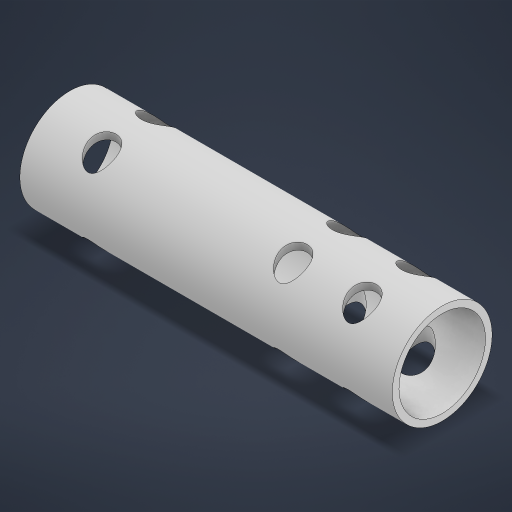
# Autodesk Inventor part: ArmSupportSteelTubing
Saved by Autodesk Inventor 2024 (Build 280153000, 153)
## iProperties
Created: 2024-02-23
Part Number: ArmSupportSteelTubing
Material: Generic
Document SubType Name: Modeling
Designer: avsar
Density: 1 g/cm^3
Appearance: Default
Author: avsar
Autodesk Inventor part; units mm, degrees
ref_plane "YZ Plane" through (0, 0, 0) normal (1, 0, 0) x (0, 1, 0)
ref_plane "XZ Plane" through (0, 0, 0) normal (0, 1, 0) x (-1, 0, 0)
sketch "Sketch1" plane through (0, 0, 0) normal (1, 0, 0) x (0, 1, 0)
  circle A0 centre (0, 0) radius 6.5
  circle A1 centre (0, 0) radius 7.5
  dimension "d0" = 13
  dimension "d1" = 15
  constraints: 2 centre point, 2 coincident
  measures "d0" diameter of A0
  measures "d1" diameter of A1
extrude "Extrusion1" add sketch "Sketch1" along normal blind 56
sketch "Sketch2" plane through (56, 0, 0) normal (1, 0, 0) x (0, 0, -1)
  circle A0 centre (0, 0) radius 7.5 construction
  line L0 (0, 7.5) -> (0, -7.5)
  constraints: 2 end point, 2 point on circle, 1 midpoint, 1 vertical
ref_plane "Work Plane1" through (56, 7.5, 0) normal (0, 1, 0) x (-1, 0, 0)
sketch "Sketch3" plane through (56, 7.5, 0) normal (0, 1, 0) x (-1, 0, 0)
  circle A0 centre (8, -4) radius 2.1
  circle A1 centre (8, 4) radius 2.1
  line L0 (8, 4) -> (8, -4) construction
  line L1 (56, -7.5) -> (0, -7.5) construction
  line L2 (28, -7.5) -> (28, 7.5) construction
  line L3 (56, 7.5) -> (0, 7.5) construction
  line L4 (12.75, 7.5) -> (3.25, 7.5) construction
  line L5 (3.25, 7.5) -> (3.25, -7.5) construction
  line L6 (3.25, -7.5) -> (12.75, -7.5) construction
  line L7 (12.75, -7.5) -> (12.75, 7.5) construction
  line L8 (12.75, 7.5) -> (3.25, -7.5) construction
  line L9 (3.25, 7.5) -> (12.75, -7.5) construction
  line L10 (13.2, -7.5) -> (13.2, 7.5) construction
  circle A2 centre (18.4, -4) radius 2.1
  circle A3 centre (18.4, 4) radius 2.1
  circle A4 centre (47.15, -4) radius 2.1
  circle A5 centre (47.15, 4) radius 2.1
  line L11 (47.15, -4) -> (47.15, 4)
  point P0 (56, 0)
  point P1 (28, 0)
  point P2 (8, 0)
  point P3 (47.15, 0)
  dimension "d4" = 4.2
  dimension "d5" = 4.2
  dimension "d6" = 20
  dimension "d7" = 8
  dimension "d8" = 9.5
  dimension "d13" = 10.4
  dimension "d14" = 28.75
  dimension "d15" = 4.2
  dimension "d16" = 4.2
  dimension "d17" = 8
  constraints: 20 end point, 7 midpoint, 6 centre point, 3 point on line, 2 horizontal alignment, 2 parallel, 2 perpendicular, 2 symmetric about line, 2 vertical, 1 horizontal, 2 other
  measures "d4" diameter of A0
  measures "d5" diameter of A1
  measures "d6" distance of point (28, 0) point (8, 0)
  measures "d7" distance of L0.start L0.end
  measures "d8" distance of L6.end L5.end
  measures "d13" distance of L0.end A2.centre
  measures "d14" horizontal distance of A2.centre point (47.15, 0)
  measures "d15" diameter of A4
  measures "d16" diameter of A5
  measures "d17" distance of L11.start L11.end
extrude "Extrusion2" cut sketch "Sketch3" against normal through all
body "Solid1"
